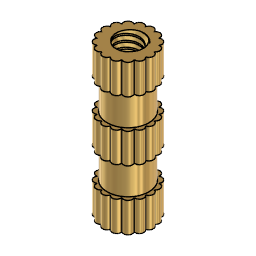
M2_10_mm_brass_thread_insert (Autodesk Fusion 360 design; units mm, degrees)
part number: 2026-06-20-09-24-02-047
Autodesk Fusion 360 part; units mm, degrees
sketch "Brass thread outline" plane through (0, 0, 0) normal (0, 0, 1) x (1, 0, 0)
  circle A0 centre (0, 0) radius 1.4
  dimension "d4" = 2.8
  constraint coincident A0.centre origin
  measures "d4" diameter of A0
extrude "Extrude1" add sketch "Brass thread outline" along normal blind 10
sketch "Ridges" plane through (0, 0, 10) normal (0, 0, 1) x (-1, 0, 0)
  circle A0 centre (0, 0) radius 1.4
  circle A1 centre (0, 0) radius 1.7
  circle A2 centre (-0.0001, -1.4) radius 0.3
  circle A3 centre (0.5357, -1.2935) radius 0.3
  circle A4 centre (0.9899, -0.99) radius 0.3
  circle A5 centre (1.2934, -0.5358) radius 0.3
  circle A6 centre (1.4, -0.0001) radius 0.3
  circle A7 centre (1.2935, 0.5357) radius 0.3
  circle A8 centre (0.99, 0.9899) radius 0.3
  circle A9 centre (0.5358, 1.2934) radius 0.3
  circle A10 centre (0.0001, 1.4) radius 0.3
  circle A11 centre (-0.5357, 1.2935) radius 0.3
  circle A12 centre (-0.9899, 0.99) radius 0.3
  circle A13 centre (-1.2934, 0.5358) radius 0.3
  circle A14 centre (-1.4, 0.0001) radius 0.3
  circle A15 centre (-1.2935, -0.5357) radius 0.3
  circle A16 centre (-0.99, -0.9899) radius 0.3
  circle A17 centre (-0.5358, -1.2934) radius 0.3
  dimension "d8" = 3.4
  dimension "d29" = 0.0001
  dimension "d31" = 360
  constraint coincident A0.centre A1.centre
  constraint coincident A0 A2.centre
  constraint tangent A1 A2
  measures "d8" diameter of A1
  measures "d29" horizontal distance of A0.centre A2.centre
extrude "Extrude2" add sketch "Ridges" against normal blind 2 contours A0 A5 A6 A7 | A0 A5 A6 A7 | A0 A6 A7 | A0 A6 A7 | A0 A5 A6 | A0 A5 A6 | A0 A6 A7 A8 | A0 A6 A7 A8 | A2 A3 A4 A5 A6 A7 A8 A9 A10 A11 A12 A13 A14 A15 A16 A17 | A0 A4 A5 A6 | A0 A4 A5 A6 | A0 A7 A8 | A0 A7 A8 | A0 A7 A8 A9 | A0 A4 A5 | A0 A4 A5 | A0 A3 A4 A5 | A0 A7 A8 A9 | A0 A8 A9 A10 | A0 A8 A9 | A0 A3 A4 A5 | A0 A2 A3 A4 | A0 A3 A4 | A0 A8 A9 | A0 A8 A9 A10 | A0 A9 A10 A11 | A0 A9 A10 | A0 A3 A4 | A0 A2 A3 A17 | A0 A2 A3 | A0 A2 A3 A4 | A0 A9 A10 | A0 A9 A10 A11 | A0 A10 A11 A12 | A0 A10 A11 | A0 A2 A3 | A0 A2 A17 | A0 A2 A16 A17 | A0 A2 A3 A17 | A0 A10 A11 | A0 A10 A11 A12 | A0 A11 A12 A13 | A0 A11 A12 | A0 A2 A16 A17 | A0 A2 A17 | A0 A15 A16 A17 | A0 A16 A17 | A0 A11 A12 | A0 A11 A12 A13 | A0 A16 A17 | A0 A15 A16 A17 | A0 A12 A13 | A0 A12 A13 | A0 A12 A13 A14 | A0 A14 A15 A16 | A0 A15 A16 | A0 A15 A16 | A0 A12 A13 A14 | A0 A14 A15 A16 | A0 A13 A14 | A0 A13 A14 | A0 A13 A14 A15 | A0 A13 A14 A15 | A0 A14 A15 | A0 A14 A15
pattern_linear "R-Pattern1" count 3 spacing 4 along (0, 0, -1) of "Extrude2"
sketch "Thread hole" plane through (0, 0, 10) normal (0, 0, 1) x (-1, 0, 0)
  circle A0 centre (0, 0) radius 1
  arc A1 (0.292, -1.4685) -> (0.8317, -1.2449) centre (0.5357, -1.2935) ccw
  arc A2 (0.8317, -1.2449) -> (1.2448, -0.8319) centre (0.9899, -0.99) ccw
  arc A3 (1.2448, -0.8319) -> (1.4684, -0.2922) centre (1.2934, -0.5358) ccw
  arc A4 (1.4684, -0.2922) -> (1.4685, 0.292) centre (1.4, -0.0001) ccw
  arc A5 (1.4685, 0.292) -> (1.2449, 0.8317) centre (1.2935, 0.5357) ccw
  arc A6 (1.2449, 0.8317) -> (0.8319, 1.2448) centre (0.99, 0.9899) ccw
  arc A7 (0.8319, 1.2448) -> (0.2922, 1.4684) centre (0.5358, 1.2934) ccw
  arc A8 (0.2922, 1.4684) -> (-0.292, 1.4685) centre (0.0001, 1.4) ccw
  arc A9 (-0.292, 1.4685) -> (-0.8317, 1.2449) centre (-0.5357, 1.2935) ccw
  arc A10 (-0.8317, 1.2449) -> (-1.2448, 0.8319) centre (-0.9899, 0.99) ccw
  arc A11 (-1.2448, 0.8319) -> (-1.4684, 0.2922) centre (-1.2934, 0.5358) ccw
  arc A12 (-1.4684, 0.2922) -> (-1.4685, -0.292) centre (-1.4, 0.0001) ccw
  arc A13 (-1.4685, -0.292) -> (-1.2449, -0.8317) centre (-1.2935, -0.5357) ccw
  arc A14 (-1.2449, -0.8317) -> (-0.8319, -1.2448) centre (-0.99, -0.9899) ccw
  arc A15 (-0.8319, -1.2448) -> (-0.2922, -1.4684) centre (-0.5358, -1.2934) ccw
  arc A16 (-0.2922, -1.4684) -> (0.292, -1.4685) centre (-0.0001, -1.4) ccw
  dimension "d11" = 2
  constraint coincident A0.centre origin
  measures "d11" diameter of A0
extrude "Extrude3" cut sketch "Thread hole" against normal blind 10 contours A0
thread "Thread1" "ISO Metric profile 2.0 M2x0.4 M2x0.4 6H" major diameter 2.074 minor diameter 1.623 pitch 0.4 angle 60 modelled right hand crest width 0.1065 on face at (-0.9988, 0.0498, 3.3333) crest through (-0.8115, 0, 9.9)
equation "outer_diameter = 2.8 mm" comment "The outer diameter of the non-ridged parts."
equation "hole_diameter = 2 mm" comment "The thread diameter of the brass insert. 2 mm for this M2 insert."
equation "height = 10 mm" comment "The height of the brass thread insert. 10 mm for this model."
equation "d4 = outer_diameter"
equation "d5 = height"
equation "ridge_diameter = 3.4 mm" comment "The outer diameter of the ridged parts."
equation "d8 = ridge_diameter"
equation "d9 = -ridge_height"
equation "d11 = hole_diameter"
equation "d12 = -height"
equation "number_of_ridges = 3" comment "The number of ridges to have along the outside."
equation "d23 = number_of_ridges"
equation "d25 = -ridge_pattern_length"
equation "ridge_pattern_length = height - ridge_height" comment "The distance to use for the rectangular pattern that repeats the ridges."
equation "ridge_height = 2 mm" comment "The height of the individual ridges."
named bodies: "M2 10 mm Brass Thread Insert"
